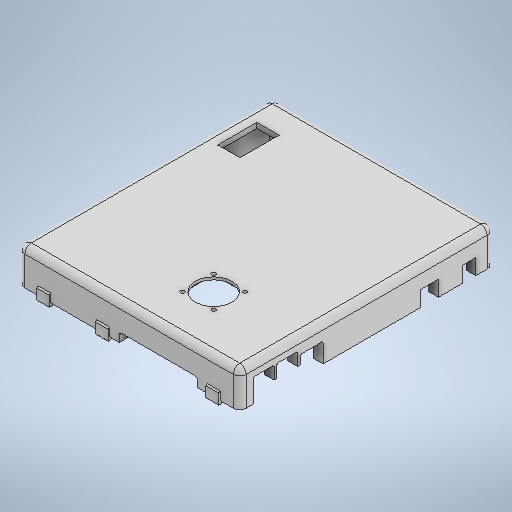
# Autodesk Inventor part: Electronic Lid 5
Saved by Autodesk Inventor 2025.2 (Build 292293000, 293)
## iProperties
Created: 2025-03-21
Part Number: Electronic Lid 5
Material: Generic
Document SubType Name: Modeling
Designer: caomi
Density: 1 g/cm^3
Appearance: Default
Author: caomi
Autodesk Inventor part; units mm, degrees
ref_plane "YZ Plane" through (0, 0, 0) normal (1, 0, 0) x (0, 1, 0)
ref_plane "XZ Plane" through (0, 0, 0) normal (0, 1, 0) x (-1, 0, 0)
ref_plane "XY Plane" through (0, 0, 0) normal (0, 0, 1) x (1, 0, 0)
sketch "Sketch1" plane through (0, 0, 0) normal (0, 1, 0) x (-1, 0, 0)
  line L0 (0, 0) -> (-155, 0)
  line L1 (-155, 0) -> (-155, 180)
  line L2 (-155, 180) -> (0, 180)
  line L3 (0, 180) -> (0, 0)
  dimension "d9" = 155
  dimension "d21" = 180
  constraints: 8 end point, 2 parallel, 1 horizontal, 1 perpendicular
  measures "d9" distance of L1.end L2.end
  measures "d21" distance of L2.end L0.start
extrude "Extrusion1" add sketch "Sketch1" along normal blind 20
shell "Shell1" thickness 7.5 outward yes removed faces 1 at (51.6667, 0, 60)
sketch "Sketch2" plane through (0, 0, 0) normal (0, -1, 0) x (1, 0, 0)
  line L0 (162.5, 187.5) -> (162.5, -7.5) projected
  line L1 (162.5, 177) -> (155, 177)
  line L2 (155, 177) -> (155, 161)
  line L3 (155, 161) -> (162.5, 161)
  line L4 (162.5, 161) -> (162.5, 177)
  line L5 (162.5, 159) -> (155, 159)
  line L6 (155, 159) -> (155, 143)
  line L7 (155, 143) -> (162.5, 143)
  line L8 (162.5, 143) -> (162.5, 159)
  line L9 (0, 180) -> (155, 180) projected
  line L10 (162.5, 141) -> (155, 141)
  line L11 (155, 141) -> (155, 123.5)
  line L12 (155, 123.5) -> (162.5, 123.5)
  line L13 (162.5, 123.5) -> (162.5, 141)
  line L14 (155, 180) -> (155, 0) projected
  line L15 (162.5, 48.5) -> (155, 48.5)
  line L16 (155, 48.5) -> (155, 34.86)
  line L17 (155, 34.86) -> (162.5, 34.86)
  line L18 (162.5, 34.86) -> (162.5, 48.5)
  line L19 (162.5, 16.5) -> (155, 16.5)
  line L20 (155, 16.5) -> (155, 6.17)
  line L21 (155, 6.17) -> (162.5, 6.17)
  line L22 (162.5, 6.17) -> (162.5, 16.5)
  line L23 (-7.5, 187.5) -> (162.5, 187.5) projected
  line L24 (130, 187.5) -> (70, 187.5)
  line L25 (70, 187.5) -> (70, 180)
  line L26 (70, 180) -> (130, 180)
  line L27 (130, 180) -> (130, 187.5)
  point P0 (158.75, 161)
  point P1 (162.5, 6.17)
  point P2 (155, 16.5)
  point P3 (162.5, 34.86)
  point P4 (155, 48.5)
  point P5 (162.5, 123.5)
  point P6 (162.5, 143)
  point P7 (162.5, 161)
  point P8 (130, 180)
  dimension "d10" = 3
  dimension "d12" = 21
  dimension "d16" = 131.5
  dimension "d18" = 163.5
  dimension "d19" = 10.33
  dimension "d20" = 13.64
  dimension "d22" = 25
  dimension "d23" = 85
  dimension "d29" = 39
  dimension "d142" = 16
  dimension "d143" = 16
  dimension "d144" = 17.5
  constraints: 48 end point, 12 parallel, 12 point on line, 6 horizontal, 6 perpendicular, 1 midpoint
  measures "d10" distance between parallel lines of L1 L9
  measures "d12" distance from line of L5 L9.end
  measures "d16" distance of L9.end L15.end
  measures "d18" distance from line of L9.end L19
  measures "d19" distance of L21.end L19.start
  measures "d20" distance of L17.end L15.start
  measures "d22" distance of L9.end L26.end
  measures "d23" distance of L9.end L25.end
  measures "d29" vertical distance of L9.end L10.start
  measures "d142" distance between parallel lines of L3 L1
  measures "d143" distance of L7.end L5.start
  measures "d144" distance from line of L10 L12.end
extrude "Board Ports" cut sketch "Sketch2" against normal blind 18 contours L0 L3 L2 L1 | L0 L7 L6 L5
extrude "Pi Power Suppply" cut sketch "Sketch2" against normal blind 7 contours L27 L9 L25 L23
fillet "Fillet4" radius 2 2 edges at (70, 7, 183.75) (130, 7, 183.75)
extrude "Extrusion10" cut sketch "Sketch2" against normal blind 8 contours L0 L5 L14 L3 | L0 L10 L14 L7
extrude "Pi Ethernet port" cut sketch "Sketch2" against normal blind 15 contours L0 L12 L11 L10
chamfer "Chamfer1" distance 1 angle 45 6 edges at (158.75, 18, 177) (158.75, 18, 161) (158.75, 18, 159) (158.75, 18, 143) (158.75, 15, 141) (158.75, 15, 123.5)
extrude "Arduino Ports" cut sketch "Sketch2" against normal blind 12 contours L0 L17 L14 L15 | L0 L21 L14 L19
fillet "Fillet1" radius 5 8 edges at (162.5, 13.75, 187.5) (-7.5, 13.75, 187.5) (162.5, 13.75, -7.5) (-7.5, 13.75, -7.5) (-7.5, 27.5, 90) (77.5, 27.5, -7.5) (77.5, 27.5, 187.5) (162.5, 27.5, 90)
fillet "Fillet6" radius 2 4 edges at (155, 10, 180) (0, 10, 180) (0, 10, 0) (155, 10, 0)
ref_plane "Work Plane6" through (142.5, 0, 177) normal (1, 0, 0) x (0, 0, -1)
ref_plane "Work Plane7" through (57.5, 0, 177) normal (1, 0, 0) x (0, 0, -1)
ref_plane "Work Plane9" through (12.5, 0, 177) normal (1, 0, 0) x (0, 0, -1)
sketch "Sketch3" plane through (162.5, 0, 95.86) normal (1, 0, 0) x (0, 0, -1)
  line L0 (-91.64, 22.5) -> (-91.64, 0) projected
  line L1 (-91.64, 0) -> (-90.84, 0)
  line L2 (-90.84, 0) -> (-90.84, -2.5)
  line L3 (-90.84, -2.5) -> (-91.64, -2.5)
  line L4 (-91.64, -2.5) -> (-91.64, 0)
  line L5 (-90.84, -2.5) -> (-89.84, -1.5)
  line L6 (-89.84, -1.5) -> (-90.84, -0.5)
  line L7 (-89.84, -1.5) -> (-90.84, -1.5) construction
  line L8 (-86.64, 22.5) -> (98.36, 22.5) projected
  line L9 (5.86, 51.3756) -> (5.86, -39.6704) construction
  line L10 (103.36, 0) -> (102.56, 0)
  line L11 (102.56, 0) -> (102.56, -2.5)
  line L12 (102.56, -2.5) -> (103.36, -2.5)
  line L13 (103.36, -2.5) -> (103.36, 0)
  line L14 (102.56, -2.5) -> (101.56, -1.5)
  line L15 (101.56, -1.5) -> (102.56, -0.5)
  line L16 (101.56, -1.5) -> (102.56, -1.5) construction
  line L17 (-91.64, -2.5) -> (-92.64, -2.5)
  line L18 (-92.64, -2.5) -> (-92.64, 5.5)
  line L19 (-92.64, 5.5) -> (-91.64, 5.5)
  line L20 (-91.64, 5.5) -> (-91.64, -2.5)
  line L21 (-92.64, 5.5) -> (-91.64, 6.5)
  circle A0 centre (-91.94, -2.5) radius 0.3
  line L22 (104.36, -2.5) -> (104.36, 5.5)
  line L23 (104.36, 5.5) -> (103.36, 5.5)
  line L24 (104.36, 5.5) -> (103.36, 6.5)
  circle A1 centre (103.66, -2.5) radius 0.3
  line L25 (103.36, -2.5) -> (104.36, -2.5)
  line L26 (103.36, 0) -> (103.36, 22.5) projected
  line L27 (103.36, 0) -> (98.36, 0) projected
  point P0 (95.86, 0)
  point P1 (5.86, 22.5)
  point P2 (-92.24, -2.5)
  point P3 (-92.2373, -2.5)
  point P4 (103.96, -2.5)
  dimension "d130" = 0.6
  dimension "d35" = 0.8
  dimension "d36" = 2.5
  dimension "d37" = 1
  dimension "d38" = 45
  dimension "d128" = 45
  dimension "d129" = 1
  dimension "d133" = 8
  constraints: 48 end point, 11 symmetric about line, 7 point on line, 4 parallel, 3 perpendicular, 2 horizontal, 1 centre point, 1 midpoint, 1 vertical, 5 other
  measures "d35" distance of L2.end L3.end
  measures "d36" distance of L3.end L0.end
  measures "d37" distance of L5.end L7.end
  measures "d38" angle of L2 L5
  measures "d128" angle of L21 L19
  measures "d129" distance between parallel lines of L20 L18
  measures "d133" distance from line of L17.end L19
extrude "Snap tab 1" add sketch "Sketch3" along normal mid plane 9.8 from surface at -20 contours L0 L19 L21 | L0 L4 A0 L17 L18 L19 | L1 L2 L3 L4 | L17 A0 | L6 L5 L2 picked at (-91.9521, -2.3078)
extrude "Snap tab 1 Groove" cut sketch "Sketch3" along normal mid plane 4 from surface at -20 contours A0 L17 | L17 A0
extrude "Snap tab 2" add sketch "Sketch3" along normal mid plane 9.8 from surface at -105 contours L0 L19 L21 | L0 L4 A0 L17 L18 L19 | L1 L2 L3 L4 | L17 A0 | L6 L5 L2 picked at (-91.9521, -2.3078)
extrude "Snap tab 2 Groove" cut sketch "Sketch3" along normal mid plane 4 from surface at -105 contours A0 L17 | L17 A0
extrude "Snap tab 3" add sketch "Sketch3" along normal mid plane 9.8 from surface at -150 contours L0 L19 L21 | L0 L4 A0 L17 L18 L19 | L1 L2 L3 L4 | L17 A0 | L6 L5 L2 picked at (-91.9521, -2.3078)
extrude "Snap tab 3 GRoove" cut sketch "Sketch3" along normal mid plane 4 from surface at -150 contours A0 L17 | L17 A0
fillet "Fillet5" radius 1 3 edges at (12.5, -1.5, 185.7) (57.5, -1.5, 185.7) (142.5, -1.5, 185.7)
ref_plane "Work Plane11" through (157.5, 0, 90) normal (0, 0, -1) x (-1, 0, 0)
mirror "Mirror1" about plane through (157.5, 0, 90) normal (0, 0, -1) of "Snap tab 1", "Snap tab 1 Groove", "Snap tab 2", "Snap tab 2 Groove", "Snap tab 3 GRoove", "Snap tab 3", "Fillet5"
sketch "Sketch4" plane through (-7.5, 7, 189.5) normal (-1, 0, 0) x (0, 0, 1)
  circle A0 centre (-24.5, -7) radius 5
  point P0 (-189.5, -7)
  point P1 (-9.5, -7)
  dimension "d67" = 10
  dimension "d145" = 15
  constraints: 1 centre point
  measures "d67" diameter of A0
  measures "d145" distance of point (-9.5, -7) A0.centre
extrude "DC terminal port" cut sketch "Sketch4" against normal up to surface (7.5 mm away)
ref_plane "Work Plane10" through (0, -7, 180) normal (0, -1, 0) x (1, 0, 0)
sketch "Sketch5" plane through (0, 0, 180) normal (0, -1, 0) x (1, 0, 0)
  line L0 (-1.5, -9.75) -> (-1.5, -20.25)
  line L1 (-1.5, -20.25) -> (11.5, -22)
  line L2 (11.5, -22) -> (11.5, -8)
  line L3 (11.5, -8) -> (-1.5, -9.75)
  line L4 (-4.6276, -15) -> (10.9018, -15) construction
  line L5 (-7.5, -182.5) -> (-7.5, 2.5) projected
  line L6 (-7.5, -20) -> (-7.5, -10) projected
  point P0 (-7.5, -15)
  dimension "d69" = 10.5
  dimension "d70" = 14
  dimension "d71" = 13
  dimension "d146" = 6
  constraints: 10 end point, 1 horizontal, 1 midpoint, 1 point on line, 1 vertical, 1 other
  measures "d69" distance of L0.start L0.end
  measures "d70" distance of L1.end L2.end
  measures "d71" distance between parallel lines of L2 L0
  measures "d146" distance between parallel lines of L5 L0
extrude "DC terminal fitting" cut sketch "Sketch5" against normal blind 3
sketch "Sketch7" plane through (0, 20, 180) normal (0, -1, 0) x (1, 0, 0)
  line L0 (4, -164.2) -> (21, -164.2)
  line L1 (21, -164.2) -> (21, -134.2)
  line L2 (21, -134.2) -> (4, -134.2)
  line L3 (4, -134.2) -> (4, -164.2)
  line L4 (155, -180) -> (0, -180) projected
  line L5 (0, -180) -> (0, 0) projected
  line L6 (84.75, -50.25) -> (115.25, -50.25)
  line L7 (115.25, -50.25) -> (115.25, -19.75)
  line L8 (115.25, -19.75) -> (84.75, -19.75)
  line L9 (84.75, -19.75) -> (84.75, -50.25)
  line L10 (53.5433, -35) -> (106.3697, -35) construction
  line L11 (100, -38.9742) -> (100, -90.2203) construction
  circle A0 centre (88, -47) radius 1.5
  circle A1 centre (88, -23) radius 1.5
  circle A2 centre (112, -47) radius 1.5
  circle A3 centre (112, -23) radius 1.5
  circle A4 centre (100, -35) radius 14
  line L12 (155, -2) -> (155, -178) projected
  line L13 (2, 0) -> (153, 0) projected
  point P0 (0, -95.4083)
  dimension "d83" = 15.8
  dimension "d84" = 45.8
  dimension "d85" = 4
  dimension "d86" = 21
  dimension "d91" = 30.5
  dimension "d92" = 30.5
  dimension "d93" = 3
  dimension "d95" = 24
  dimension "d96" = 24
  dimension "d101" = 28
  dimension "d149" = 55
  dimension "d150" = 35
  constraints: 20 end point, 5 centre point, 4 parallel, 3 horizontal, 3 symmetric about line, 2 perpendicular, 2 point on line, 1 vertical, 5 other
  measures "d83" distance between parallel lines of L4 L0
  measures "d84" distance from line of L4 L2.end
  measures "d85" distance between parallel lines of L5 L3
  measures "d86" distance between parallel lines of L5 L1
  measures "d91" distance of L6.end L7.end
  measures "d92" distance of L6.start L6.end
  measures "d93" diameter of A0
  measures "d95" distance of A3.centre A2.centre
  measures "d96" distance of A2.centre A0.centre
  measures "d101" diameter of A4
  measures "d149" distance from line of L12 A4.centre
  measures "d150" distance from line of L13 A4.centre
extrude "Motor driver heat sink hole" cut sketch "Sketch7" against normal blind 20 contours L3 L2 L1 L0
sketch "Sketch8" plane through (0, 20, 180) normal (0, -1, 0) x (1, 0, 0)
  line L0 (4, -134.2) -> (21, -134.2) projected
  line L1 (21, -134.2) -> (21, -164.2) projected
  line L2 (21, -164.2) -> (4, -164.2) projected
  line L3 (4, -164.2) -> (4, -134.2) projected
  line L4 (0, 0) -> (155, 0) projected
  line L5 (0, -180) -> (0, 0) projected
  line L6 (0, -92.3585) -> (0, -87.6415) projected
  line L7 (0, -180) -> (0, 0) projected
  line L8 (155, -180) -> (0, -180) projected
  line L9 (155, 0) -> (155, -180) projected
extrude "Base thinning" cut sketch "Sketch8" against normal blind 3.5
extrude "Fan recess face" cut sketch "Sketch7" against normal blind 2 from surface at -3.5 contours L9 L8 L7 L6 | A0 | A1 | A2 | A3 | A4
extrude "Fan mounting holes" cut sketch "Sketch7" against normal through all contours A0 | A1 | A2 | A3
extrude "Fan opening" cut sketch "Sketch7" against normal blind 10 contours A4
sketch "Sketch10" plane through (-7.5, 0, 182.5) normal (-1, 0, 0) x (0, 0, 1)
  line L0 (-185, 0) -> (0, 0) projected
  line L1 (-185, 0) -> (0, 0) projected
  line L2 (-67.5, 12) -> (-117.5, 12) construction
  line L3 (-67.5, 20) -> (-117.5, 20)
  line L4 (-117.5, 4) -> (-67.5, 4)
  arc A0 (-67.5, 4) -> (-67.5, 20) centre (-67.5, 12) ccw
  arc A1 (-117.5, 20) -> (-117.5, 4) centre (-117.5, 12) ccw
  point P0 (-101.95, 0)
  point P1 (-99.15, 0)
  point P2 (-69.95, 0)
  point P3 (-182.5, 0)
  point P4 (-92.5, 12)
  point P5 (-92.5, 0)
  dimension "d118" = 50
  dimension "d119" = 8
  dimension "d120" = 12
  constraints: 8 end point, 4 point on circle, 4 tangent, 2 centre point, 2 midpoint, 1 horizontal, 1 parallel, 1 vertical alignment
  measures "d118" distance of L2.start L2.end
  measures "d119" radius of A1
  measures "d120" distance between parallel lines of L1 L2
extrude "Extra cable slot" cut sketch "Sketch10" against normal blind 10
equation "\"d92\" = d91"
equation "\"d96\" = d95"
body "Solid1"
